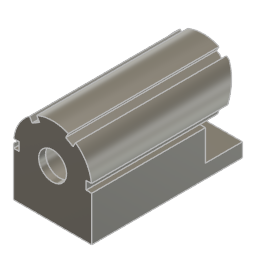
some random stuff (Autodesk Fusion 360 design; units mm, degrees)
Autodesk Fusion 360 part; units mm, degrees
sketch "Sketch1" plane through (0, 0, 0) normal (0, 0, 1) x (1, 0, 0)
  line L0 (0, 0) -> (-56, 0)
  line L1 (-56, 0) -> (-56, 35)
  line L2 (0, 35) -> (0, 0)
  line L3 (-56, 0) -> (-28, 0)
  circle A0 centre (-28, 35) radius 10
  line L4 (-28, 0) -> (-4, 0)
  line L5 (-28, 35) -> (0, 35) construction
  line L6 (-28, 35) -> (-28, 0) construction
  line L7 (-4, 0) -> (-4, 35) construction
  line L8 (0, 35) -> (0, 32)
  line L9 (0, 32) -> (-4, 32)
  line L10 (-4, 32) -> (-4, 38)
  line L11 (-4, 38) -> (-0.1612, 38)
  line L12 (0, 35) -> (0, 32)
  line L13 (-28, 35) -> (-14, 59.2487) construction
  line L14 (-28, 35) -> (-42, 59.2487) construction
  line L15 (-28, 35) -> (-56, 35) construction
  line L16 (-18.5981, 57.2846) -> (-16.6787, 60.6091)
  line L17 (-11.4825, 57.6091) -> (-13.4019, 54.2846)
  line L18 (-13.4019, 54.2846) -> (-18.5981, 57.2846)
  line L19 (-42.5981, 54.2846) -> (-44.5175, 57.6091)
  line L20 (-39.3213, 60.6091) -> (-37.4019, 57.2846)
  line L21 (-37.4019, 57.2846) -> (-42.5981, 54.2846)
  line L22 (-52, 32) -> (-55.8388, 32)
  line L23 (-55.8388, 38) -> (-52, 38)
  line L24 (-52, 38) -> (-52, 32)
  line L25 (-44.5981, 12.2513) -> (-44.5175, 12.3909)
  arc A1 (-0.1612, 32) -> (-42, 59.2487) centre (-28, 35) ccw
  line L26 (-16.5981, 9.2513) -> (-16.6787, 9.3909)
  arc A2 (0, 35) -> (-11.4825, 57.6091) centre (-28, 35) ccw
  arc A3 (-14, 59.2487) -> (-56, 35) centre (-28, 35) ccw
  arc A4 (-56, 35) -> (-55.8388, 32) centre (-28, 35) ccw
  arc A5 (-42, 59.2487) -> (-55.8388, 32) centre (-28, 35) ccw
  arc A6 (-14, 59.2487) -> (-55.8388, 32) centre (-28, 35) ccw
  arc A7 (-0.1612, 32) -> (0, 35) centre (-28, 35) ccw
  arc A8 (-0.1612, 32) -> (-14, 59.2487) centre (-28, 35) ccw
  circle A9 centre (-28, 35) radius 15
  dimension "d1" = 56
  dimension "d2" = 35
  dimension "d3" = 20
  dimension "d4" = 24
  dimension "d5" = 3
  dimension "d7" = 60
  dimension "d8" = 60
  dimension "d13" = 30
  constraint horizontal L0
  constraint vertical L1
  constraint vertical L2
  constraint coincident L0.start L2.end
  constraint midpoint L0 L3.end
  constraint concentric A0 A2
  constraint parallel L0 L4
  constraint coincident A0.centre L5.start
  constraint perpendicular L2 L5
  constraint perpendicular L0 L6
  constraint coincident L5 L7.end
  constraint perpendicular L5 L7
  constraint perpendicular L5 L8
  constraint horizontal L9
  constraint vertical L10
  constraint horizontal L11
  constraint vertical L12
  constraint coincident L11.end A2
  constraint coincident L13.end A2
  constraint coincident L14.end A2
  constraint perpendicular L6 L15
  constraint coincident L25.end A6
  constraint coincident L26.end A5
  constraint concentric A2 A3
  constraint coincident L20.start A6
  constraint coincident L23.start A6
  constraint coincident L9 A1.start
  constraint concentric A4 A9
  measures "d1" distance of L0.start L0.end
  measures "d2" distance of L0.start L2.start
  measures "d3" diameter of A0
  measures "d4" distance of L3.end L4.end
  measures "d5" distance of L2.start L8.end
  measures "d7" angle of L5 L13
  measures "d8" angle of L13 L14
  measures "d13" diameter of A9
extrude "Extrude1" add sketch "Sketch1" against normal blind 108 contours L0 L1 L2 L3 L4 L9 L10 L11 L16 L17 L18 L19 L20 L21 L22 L23 L24 A1 A2 A3 A4 A5 A6 A8
sketch "Sketch2" plane through (0, 0, 0) normal (1, 0, 0) x (0, 0, -1)
  line L0 (0, 32) -> (0, 0)
  line L1 (0, 0) -> (108, 0)
  line L2 (108, 0) -> (108, 32)
  line L3 (108, 32) -> (0, 32)
  line L4 (108, 0) -> (108, 56)
  line L5 (108, 56) -> (81.4419, 10)
  line L6 (108, 0) -> (108, 10)
  line L7 (108, 10) -> (81.4419, 10)
  dimension "d16" = 56
  dimension "d17" = 30
  dimension "d18" = 10
  constraint coincident L1.end L2.start
  constraint perpendicular L1 L4
  constraint perpendicular L1 L6
  constraint perpendicular L4 L7
  measures "d16" distance of L1.end L4.end
  measures "d17" angle of L4 L5
  measures "d18" distance of L1.end L6.end
extrude "Extrude2" cut sketch "Sketch2" against normal blind 130 contours L3 L4 L5 | L2 L3 L4 L5 L7
sketch "Sketch3" plane through (0, 0, 0) normal (1, 0, 0) x (0, 0, -1)
  line L0 (81.4419, 10) -> (94.1436, 32)
  line L1 (94.1436, 32) -> (0, 32)
  line L2 (0, 32) -> (0, 0)
  line L3 (0, 0) -> (108, 0)
  line L4 (108, 0) -> (108, 10)
  line L5 (108, 10) -> (81.4419, 10)
  line L6 (81.4419, 10) -> (81.4419, 32)
  line L7 (81.4419, 32) -> (94.1436, 32)
  line L8 (94.1436, 32) -> (81.4419, 10)
  constraint coincident L0.start L5.end
  constraint coincident L1 L6.end
  constraint perpendicular L1 L6
  constraint coincident L0.end L1.start
extrude "Extrude3" cut sketch "Sketch3" against normal blind 140 contours L0 L1 L6 L7 L8
sketch "Sketch4" plane through (0, 0, 0) normal (0, 0, 1) x (1, 0, 0)
  circle A0 centre (-28, 35) radius 15
  line L0 (-56, 0) -> (0, 0)
  line L1 (0, 0) -> (0, 32)
  line L2 (0, 32) -> (-4, 32)
  line L3 (-4, 32) -> (-4, 38)
  line L4 (-4, 38) -> (-0.1612, 38)
  arc A1 (-0.1612, 38) -> (-11.4825, 57.6091) centre (-28, 35) ccw
  line L5 (-11.4825, 57.6091) -> (-13.4019, 54.2846)
  line L6 (-13.4019, 54.2846) -> (-18.5981, 57.2846)
  line L7 (-18.5981, 57.2846) -> (-16.6787, 60.6091)
  arc A2 (-16.6787, 60.6091) -> (-39.3213, 60.6091) centre (-28, 35) ccw
  line L8 (-39.3213, 60.6091) -> (-37.4019, 57.2846)
  line L9 (-37.4019, 57.2846) -> (-42.5981, 54.2846)
  line L10 (-42.5981, 54.2846) -> (-44.5175, 57.6091)
  arc A3 (-44.5175, 57.6091) -> (-55.8388, 38) centre (-28, 35) ccw
  line L11 (-55.8388, 38) -> (-52, 38)
  line L12 (-52, 38) -> (-52, 32)
  line L13 (-52, 32) -> (-55.8388, 32)
  arc A4 (-56, 35) -> (-55.8388, 32) centre (-28, 35) ccw
  line L14 (-56, 35) -> (-56, 0)
  circle A5 centre (-28, 35) radius 10
  dimension "d23" = 20
  constraint concentric A0 A5
  measures "d23" diameter of A5
extrude "Extrude4" add sketch "Sketch4" against normal blind 5 contours A0
